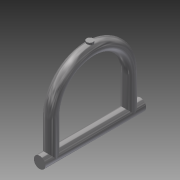
# Autodesk Inventor part: 0D
Saved by Autodesk Inventor 2014 (Build 180170000, 170)
## iProperties
Company: HERA Project
Created: 2013-12-04
Part Number: 0D
Material: Stainless Steel
Document SubType Name: Modeling
Designer: Dave
Mass: 20.3859 g
Surface Area: 19.9275 cm^2
Volume: 2.52301 cm^3
Density: 8.08 g/cm^3
Description: anchor D for feed
Appearance: Semi-Polished
Author: David DeBoer
Autodesk Inventor part; units mm, degrees
ref_plane "YZ Plane" through (0, 0, 0) normal (1, 0, 0) x (0, 1, 0)
ref_plane "XZ Plane" through (0, 0, 0) normal (0, 1, 0) x (-1, 0, 0)
ref_plane "XY Plane" through (0, 0, 0) normal (0, 0, 1) x (1, 0, 0)
sketch "Sketch1" plane through (0, 0, 0) normal (0, 0, 1) x (1, 0, 0)
  circle A0 centre (0, 0) radius 2.54
  dimension "d0" = 5.08
  constraints: 1 centre point, 1 coincident
  measures "d0" diameter of A0
extrude "Extrusion1" add sketch "Sketch1" along normal blind 44.45
sketch "Sketch2" plane through (0, 0, 44.45) normal (0, 0, 1) x (1, 0, 0)
  circle A0 centre (0, 0) radius 2.54 projected
  point P0 (0, 2.54)
  constraints: 1 vertical alignment, 1 other
ref_plane "Work Plane1" through (0, 2.54, 44.45) normal (0, 1, 0) x (-1, 0, 0)
sketch "Sketch3" plane through (0, 2.54, 44.45) normal (0, 1, 0) x (-1, 0, 0)
  circle A0 centre (0, -39.37) radius 2.54
  circle A1 centre (0, -5.08) radius 2.54
  line L0 (2.54, 0) -> (-2.54, 0) projected
  point P0 (0, -44.45)
  dimension "d4" = 5.08
  dimension "d6" = 5.08
  dimension "d7" = 5.08
  dimension "d8" = 5.08
  constraints: 2 centre point
  measures "d4" diameter of A0
  measures "d6" distance of point (0, -44.45) A0.centre
  measures "d7" diameter of A1
  measures "d8" distance from line of A1.centre L0
extrude "Extrusion2" add sketch "Sketch3" along normal blind 12.7 and the other way blind 2.54
sketch "Sketch4" plane through (0, 15.24, 39.37) normal (0, 1, 0) x (1, 0, 0)
  circle A0 centre (0, 0) radius 2.54 projected
  line L0 (0, 0) -> (0, 34.29) construction
  line L1 (0, 17.145) -> (4.1545, 17.145) construction
  point P0 (0, 39.37)
  dimension "d14" = 34.29
  constraints: 4 end point, 1 midpoint, 1 perpendicular
  measures "d14" distance of L0.start L0.end
revolve "Revolution1" add sketch "Sketch4" angle 180 about axis through (0, 15.24, 22.225) along (-1, 0, 0)
ref_plane "Work Plane3" through (0, 33.02, 44.45) normal (0, 1, 0) x (-1, 0, 0)
sketch "Sketch6" plane through (0, 33.02, 44.45) normal (0, 1, 0) x (-1, 0, 0)
  circle A0 centre (0, -22.1526) radius 1.449
  point P0 (0, -44.45)
  constraints: 1 centre point
extrude "Extrusion3" add sketch "Sketch6" along normal blind 2.54
body "Solid1"
